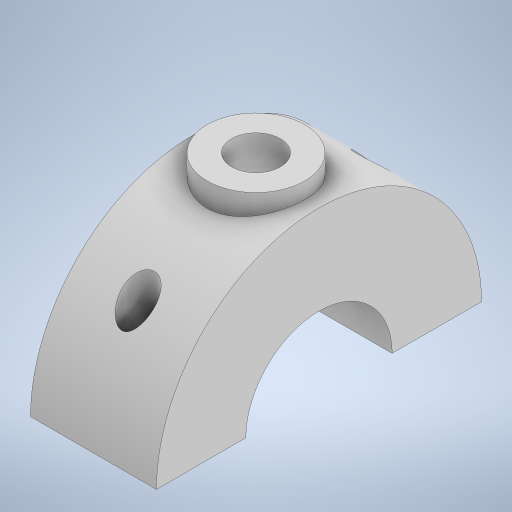
# Autodesk Inventor part: Parte1
Saved by Autodesk Inventor 2023 (Build 270158000, 158)
## iProperties
Created: 2022-11-03
Part Number: Parte1
Material: Generic
Document SubType Name: Modeling
Designer: ivanm
Density: 1 g/cm^3
Appearance: Default
Author: ivanm
Autodesk Inventor part; units mm, degrees
sketch "Sketch1" plane through (0, 0, 0) normal (1, 0, 0) x (0, 1, 0)
  arc A0 (0, -9) -> (0, 9) centre (0, 0) ccw
  arc A1 (0, -20) -> (0, 20) centre (0, 0) ccw
  line L0 (0, 20) -> (0, 9)
  line L1 (0, -9) -> (0, -20)
  dimension "d0" = 18
  dimension "d1" = 40
  dimension "d23" = 11
  dimension "d24" = 11
  constraints: 4 end point, 4 point on circle, 3 coincident, 2 centre point, 2 vertical
  measures "d0" diameter of A0
  measures "d1" diameter of A1
  measures "d23" distance of L0.start L0.end
  measures "d24" distance of L1.start L1.end
extrude "Extrusion1" add sketch "Sketch1" along normal blind 15.5
ref_plane "Work Plane1" through (0, 20, 0) normal (0, -1, 0) x (1, 0, 0)
sketch "Sketch2" plane through (0, 20, 0) normal (0, -1, 0) x (1, 0, 0)
  line L0 (0, -20) -> (0, 20) projected
  line L1 (0, 20) -> (15.5, 20) projected
  line L2 (15.5, -20) -> (15.5, 20) projected
  line L3 (0, -20) -> (15.5, -20) projected
  line L4 (0, 0) -> (15.5, 0) construction
  line L5 (7.75, -20) -> (7.75, 20) construction
  circle A0 centre (7.75, 0) radius 6
  circle A1 centre (7.75, 0) radius 3
  dimension "d6" = 6
  dimension "d7" = 12
  constraints: 4 end point, 4 midpoint, 2 centre point, 1 coincident, 1 perpendicular
  measures "d6" diameter of A1
  measures "d7" diameter of A0
extrude "Extrusion2" add sketch "Sketch2" along normal up to surface contours A0
extrude "Extrusion3" add sketch "Sketch2" against normal blind 2 contours A0
extrude "Extrusion4" cut sketch "Sketch2" along normal through all contours A1
ref_plane "Work Plane2" through (0, -9, 0) normal (0, -1, 0) x (1, 0, 0)
sketch "Sketch3" plane through (0, -9, 0) normal (0, -1, 0) x (1, 0, 0)
  spline S0 degree 5 poles (10.75, 0) (10.75, 0.1919) (10.7347, 0.3833) (10.7041, 0.5714) (10.6596, 0.7535) (10.4814, 1.3019) (10.3046, 1.6367) (10.089, 1.9249) (9.8507, 2.1665) (9.2646, 2.6229) (8.9063, 2.8107) (8.5304, 2.9351) (8.1467, 2.9984) (7.377, 3.0016) (6.9919, 2.9412) (6.6144, 2.8193) (6.2543, 2.6338) (5.7403, 2.2393) (5.5662, 2.0777) (5.4035, 1.894) (5.2559, 1.6877) (5.0482, 1.3144) (4.976, 1.1609) (4.9132, 0.9991) (4.8615, 0.8299) (4.7677, 0.4104) (4.7372, 0.1545) (4.7351, -0.1058) (4.7615, -0.3627) (4.8805, -0.9373) (4.9926, -1.2464) (5.1398, -1.524) (5.3101, -1.7687) (5.6345, -2.1369) (5.7791, -2.275) (5.9315, -2.3978) (6.09, -2.5059) (6.5339, -2.7615) (6.8293, -2.8812) (7.1334, -2.9604) (7.4415, -3) (8.1364, -3) (8.5223, -2.9377) (8.9004, -2.8136) (9.2609, -2.6254) (9.7711, -2.2286) (9.9417, -2.0687) (10.1012, -1.8873) (10.2462, -1.6839) (10.5091, -1.2113) (10.6251, -0.9341) (10.7077, -0.6337) (10.75, -0.3188) (10.75, 0) knots 0 0 0 0 0 0 0.042119 0.042119 0.042119 0.042119 0.133094 0.133094 0.133094 0.133094 0.249329 0.249329 0.249329 0.249329 0.365878 0.365878 0.365878 0.365878 0.430395 0.430395 0.430395 0.430395 0.47098 0.47098 0.47098 0.47098 0.5274 0.5274 0.5274 0.5274 0.602942 0.602942 0.602942 0.602942 0.657091 0.657091 0.657091 0.657091 0.750295 0.750295 0.750295 0.750295 0.867023 0.867023 0.867023 0.867023 0.930426 0.930426 0.930426 0.930426 1 1 1 1 1 1 projected
  line L0 (0, 9) -> (0, -9) projected
  line L1 (0, -9) -> (15.5, -9) projected
  line L2 (15.5, 9) -> (15.5, -9) projected
  line L3 (0, 9) -> (15.5, 9) projected
  circle A0 centre (7.75, 0) radius 3 projected
  circle A1 centre (7.75, 0) radius 5
  point P0 (0, 0)
  dimension "d14" = 10
  constraints: 1 centre point, 1 coincident, 1 vertical alignment, 1 other
  measures "d14" diameter of A1
extrude "Extrusion5" cut sketch "Sketch3" against normal blind 20.4 contours A1
ref_plane "Work Plane3" through (0, -20, 0) normal (0, -1, 0) x (1, 0, 0)
sketch "Sketch4" plane through (0, -20, 0) normal (0, -1, 0) x (1, 0, 0)
  line L0 (0, 20) -> (0, 9) projected
  line L1 (0, 9) -> (15.5, 9) projected
  line L2 (15.5, 20) -> (15.5, 9) projected
  line L3 (0, 20) -> (15.5, 20) projected
  line L4 (0, -9) -> (0, -20) projected
  line L5 (0, -20) -> (15.5, -20) projected
  line L6 (15.5, -9) -> (15.5, -20) projected
  line L7 (0, -9) -> (15.5, -9) projected
  circle A0 centre (7.75, 14.5) radius 2
  circle A1 centre (7.75, -14.5) radius 2
  line L8 (15.5, 14.5) -> (0, 14.5) construction
  line L9 (7.75, 9) -> (7.75, 20) construction
  line L10 (7.75, -20) -> (7.75, -9) construction
  line L11 (15.5, -14.5) -> (0, -14.5) construction
  point P0 (0, 0)
  dimension "d19" = 4
  dimension "d20" = 4
  constraints: 10 midpoint, 8 end point, 2 centre point, 2 coincident
  measures "d19" diameter of A0
  measures "d20" diameter of A1
extrude "Extrusion6" cut sketch "Sketch4" against normal through all contours A0 | A1
equation "\"d24\" = d23"
equation "\"d20\" = d19"
body "Solid1"
